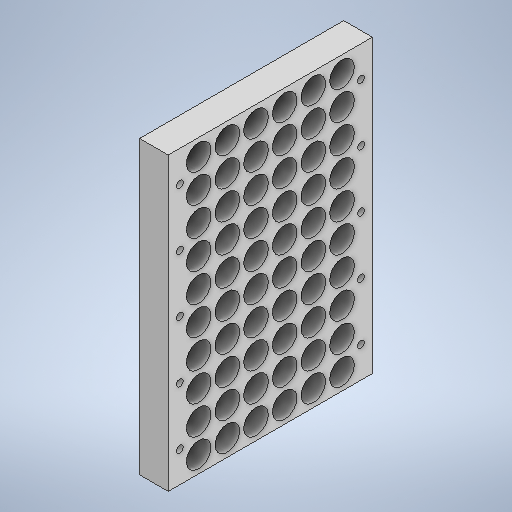
# Autodesk Inventor part: Battery Holder pt2
Saved by Autodesk Inventor 2025.2 (Build 292293000, 293)
## iProperties
Created: 2025-03-23
Part Number: Battery Holder pt2
Material: Generic
Document SubType Name: Modeling
Designer: Mathias B. Kampp
Density: 1 g/cm^3
Appearance: Default
Author: Mathias B. Kampp
## iProperties of the stored document Battery Holder pt2_3DPrint.ipt
Created: 2025-03-24
Part Number: Battery Holder pt2_3DPrint
Material: Generic
Document SubType Name: Modeling
Designer: Mathias B. Kampp
Density: 1 g/cm^3
Appearance: Default
Author: Mathias B. Kampp
Autodesk Inventor part; units mm, degrees
ref_plane "YZ Plane" through (0, 0, 0) normal (1, 0, 0) x (0, 1, 0)
ref_plane "XZ Plane" through (0, 0, 0) normal (0, 1, 0) x (-1, 0, 0)
ref_plane "XY Plane" through (0, 0, 0) normal (0, 0, 1) x (1, 0, 0)
sketch "Sketch1" plane through (0, 0, 0) normal (1, 0, 0) x (0, 1, 0)
  line L0 (0, 0) -> (0, -178)
  line L1 (0, -178) -> (254, -178)
  line L2 (254, -178) -> (254, 0)
  line L3 (254, 0) -> (0, 0)
  circle A0 centre (14.5, -26.5) radius 10.7
  circle A1 centre (39.5, -26.5) radius 10.7
  circle A2 centre (64.5, -26.5) radius 10.7
  circle A3 centre (89.5, -26.5) radius 10.7
  circle A4 centre (114.5, -26.5) radius 10.7
  circle A5 centre (139.5, -26.5) radius 10.7
  circle A6 centre (164.5, -26.5) radius 10.7
  circle A7 centre (189.5, -26.5) radius 10.7
  circle A8 centre (214.5, -26.5) radius 10.7
  circle A9 centre (239.5, -26.5) radius 10.7
  circle A10 centre (14.5, -51.5) radius 10.7
  circle A11 centre (39.5, -51.5) radius 10.7
  circle A12 centre (64.5, -51.5) radius 10.7
  circle A13 centre (89.5, -51.5) radius 10.7
  circle A14 centre (114.5, -51.5) radius 10.7
  circle A15 centre (139.5, -51.5) radius 10.7
  circle A16 centre (164.5, -51.5) radius 10.7
  circle A17 centre (189.5, -51.5) radius 10.7
  circle A18 centre (214.5, -51.5) radius 10.7
  circle A19 centre (239.5, -51.5) radius 10.7
  circle A20 centre (14.5, -76.5) radius 10.7
  circle A21 centre (39.5, -76.5) radius 10.7
  circle A22 centre (64.5, -76.5) radius 10.7
  circle A23 centre (89.5, -76.5) radius 10.7
  circle A24 centre (114.5, -76.5) radius 10.7
  circle A25 centre (139.5, -76.5) radius 10.7
  circle A26 centre (164.5, -76.5) radius 10.7
  circle A27 centre (189.5, -76.5) radius 10.7
  circle A28 centre (214.5, -76.5) radius 10.7
  circle A29 centre (239.5, -76.5) radius 10.7
  circle A30 centre (14.5, -101.5) radius 10.7
  circle A31 centre (39.5, -101.5) radius 10.7
  circle A32 centre (64.5, -101.5) radius 10.7
  circle A33 centre (89.5, -101.5) radius 10.7
  circle A34 centre (114.5, -101.5) radius 10.7
  circle A35 centre (139.5, -101.5) radius 10.7
  circle A36 centre (164.5, -101.5) radius 10.7
  circle A37 centre (189.5, -101.5) radius 10.7
  circle A38 centre (214.5, -101.5) radius 10.7
  circle A39 centre (239.5, -101.5) radius 10.7
  circle A40 centre (14.5, -126.5) radius 10.7
  circle A41 centre (39.5, -126.5) radius 10.7
  circle A42 centre (64.5, -126.5) radius 10.7
  circle A43 centre (89.5, -126.5) radius 10.7
  circle A44 centre (114.5, -126.5) radius 10.7
  circle A45 centre (139.5, -126.5) radius 10.7
  circle A46 centre (164.5, -126.5) radius 10.7
  circle A47 centre (189.5, -126.5) radius 10.7
  circle A48 centre (214.5, -126.5) radius 10.7
  circle A49 centre (239.5, -126.5) radius 10.7
  circle A50 centre (14.5, -151.5) radius 10.7
  circle A51 centre (39.5, -151.5) radius 10.7
  circle A52 centre (64.5, -151.5) radius 10.7
  circle A53 centre (89.5, -151.5) radius 10.7
  circle A54 centre (114.5, -151.5) radius 10.7
  circle A55 centre (139.5, -151.5) radius 10.7
  circle A56 centre (164.5, -151.5) radius 10.7
  circle A57 centre (189.5, -151.5) radius 10.7
  circle A58 centre (214.5, -151.5) radius 10.7
  circle A59 centre (239.5, -151.5) radius 10.7
  circle A60 centre (27, -10) radius 3
  circle A61 centre (77, -10) radius 3
  circle A62 centre (127, -10) radius 3
  circle A63 centre (177, -10) radius 3
  circle A64 centre (227, -10) radius 3
  circle A65 centre (27, -168) radius 3
  circle A66 centre (77, -168) radius 3
  circle A67 centre (127, -168) radius 3
  circle A68 centre (177, -168) radius 3
  circle A69 centre (227, -168) radius 3
  dimension "d0" = 178
  dimension "d1" = 254
  dimension "d2" = 21.4
  dimension "d5" = 25
  dimension "d8" = 25
  dimension "d11" = 6
  dimension "d14" = 50
  dimension "d17" = 158
  constraints: 70 centre point, 8 end point, 3 perpendicular, 3 vertical, 2 horizontal, 136 other
  measures "d0" distance of L0.start L0.end
  measures "d1" distance of L0.end L1.end
  measures "d2" diameter of A0
  measures "d5" distance of A0.centre A1.centre
  measures "d8" distance of A0.centre A10.centre
  measures "d11" diameter of A60
  measures "d14" distance of A60.centre A61.centre
  measures "d17" distance of A60.centre A65.centre
extrude "Extrusion1" add sketch "Sketch1" along normal blind 20
sketch "Sketch2" plane through (0, 0, 0) normal (-1, 0, 0) x (0, 0, 1)
  line L0 (0, 254) -> (0, 0) projected
  line L1 (0, 0) -> (0, 254)
  line L2 (0, 254) -> (-178, 254)
  line L3 (-178, 254) -> (-178, 0)
  line L4 (-178, 0) -> (0, 0)
  line L5 (-161, 5) -> (-92, 5)
  line L6 (-92, 5) -> (-92, 24)
  line L7 (-92, 24) -> (-161, 24)
  line L8 (-161, 24) -> (-161, 5)
  line L9 (-161, 30.0755) -> (-92, 30.0755)
  line L10 (-92, 30.0755) -> (-92, 74.0755)
  line L11 (-92, 74.0755) -> (-161, 74.0755)
  line L12 (-161, 74.0755) -> (-161, 30.0755)
  line L13 (-161, 230) -> (-17, 230)
  line L14 (-17, 230) -> (-17, 249)
  line L15 (-17, 249) -> (-161, 249)
  line L16 (-161, 249) -> (-161, 230)
  line L17 (-86, 24) -> (-86, 5)
  line L18 (-86, 5) -> (-17, 5)
  line L19 (-17, 5) -> (-17, 24)
  line L20 (-17, 24) -> (-86, 24)
  line L21 (-86, 74.0755) -> (-86, 30.0755)
  line L22 (-86, 30.0755) -> (-17, 30.0755)
  line L23 (-17, 30.0755) -> (-17, 74.0755)
  line L24 (-17, 74.0755) -> (-86, 74.0755)
  line L25 (-161, 124.0755) -> (-161, 80.0755)
  line L26 (-161, 80.0755) -> (-92, 80.0755)
  line L27 (-92, 80.0755) -> (-92, 124.0755)
  line L28 (-92, 124.0755) -> (-161, 124.0755)
  line L29 (-86, 124.0755) -> (-86, 80.0755)
  line L30 (-86, 80.0755) -> (-17, 80.0755)
  line L31 (-17, 80.0755) -> (-17, 124.0755)
  line L32 (-17, 124.0755) -> (-86, 124.0755)
  line L33 (-161, 174.0755) -> (-161, 130.0755)
  line L34 (-161, 130.0755) -> (-92, 130.0755)
  line L35 (-92, 130.0755) -> (-92, 174.0755)
  line L36 (-92, 174.0755) -> (-161, 174.0755)
  line L37 (-86, 174.0755) -> (-86, 130.0755)
  line L38 (-86, 130.0755) -> (-17, 130.0755)
  line L39 (-17, 130.0755) -> (-17, 174.0755)
  line L40 (-17, 174.0755) -> (-86, 174.0755)
  line L41 (-161, 224.0755) -> (-161, 180.0755)
  line L42 (-161, 180.0755) -> (-92, 180.0755)
  line L43 (-92, 180.0755) -> (-92, 224.0755)
  line L44 (-92, 224.0755) -> (-161, 224.0755)
  line L45 (-86, 224.0755) -> (-86, 180.0755)
  line L46 (-86, 180.0755) -> (-17, 180.0755)
  line L47 (-17, 180.0755) -> (-17, 224.0755)
  line L48 (-17, 224.0755) -> (-86, 224.0755)
  circle A0 centre (-168, 27) radius 3 projected
  circle A1 centre (-168, 27) radius 3
  circle A2 centre (-10, 27) radius 3
  circle A3 centre (-168, 77) radius 3
  circle A4 centre (-10, 77) radius 3
  circle A5 centre (-168, 127) radius 3
  circle A6 centre (-10, 127) radius 3
  circle A7 centre (-168, 177) radius 3
  circle A8 centre (-10, 177) radius 3
  circle A9 centre (-168, 227) radius 3
  circle A10 centre (-10, 227) radius 3
  dimension "d22" = 178
  dimension "d23" = 69
  dimension "d24" = 19
  dimension "d25" = 44
  dimension "d26" = 144
  dimension "d27" = 19
  dimension "d30" = 75
  dimension "d37" = 75
  dimension "d40" = 50
  dimension "d45" = 158
  dimension "d48" = 50
  constraints: 96 end point, 10 centre point, 7 equal length, 6 horizontal, 6 perpendicular, 2 point on line, 2 vertical, 1 coincident, 83 other
  measures "d22" distance of L0.start L2.end
  measures "d23" distance of L7.end L6.end
  measures "d24" distance of L6.end L5.end
  measures "d25" distance of L10.end L9.end
  measures "d26" distance of L15.end L14.end
  measures "d27" distance of L14.end L13.end
  measures "d30" distance of L7.end L17.start
  measures "d37" distance of L11.end L21.start
  measures "d40" distance of L11.end L25.start
  measures "d45" distance of A1.centre A2.centre
  measures "d48" distance of A1.centre A3.centre
extrude "Extrusion2" add sketch "Sketch2" along normal blind 5
body "Solid1"
